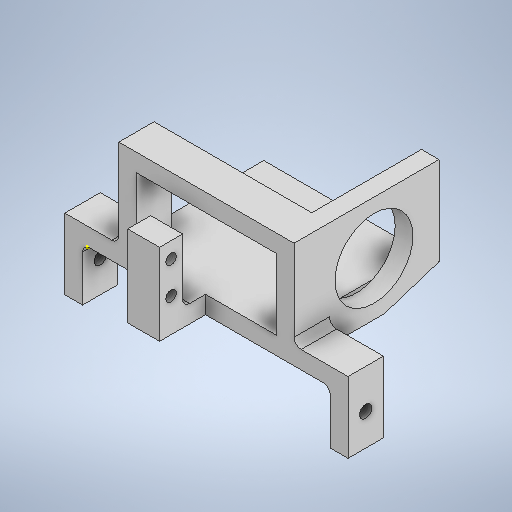
# Autodesk Inventor part: miau miau ggua gua loro loro
Saved by Autodesk Inventor 2025.2 (Build 292293000, 293)
## iProperties
Created: 2025-04-23
Part Number: miau miau ggua gua loro loro
Material: Generic
Document SubType Name: Modeling
Designer: maqmat
Density: 1 g/cm^3
Appearance: Default
Author: maqmat
Autodesk Inventor part; units mm, degrees
ref_plane "YZ Plane" through (0, 0, 0) normal (1, 0, 0) x (0, 1, 0)
ref_plane "XZ Plane" through (0, 0, 0) normal (0, 1, 0) x (-1, 0, 0)
ref_plane "XY Plane" through (0, 0, 0) normal (0, 0, 1) x (1, 0, 0)
sketch "Sketch1" plane through (0, 0, 0) normal (0, 1, 0) x (-1, 0, 0)
  line L0 (1.443, 4.6996) -> (-68.557, 4.6996)
  line L1 (-68.557, 4.6996) -> (-68.557, -5.3004)
  line L2 (-68.557, -5.3004) -> (1.443, -5.3004)
  line L3 (1.443, -5.3004) -> (1.443, 4.6996)
  line L4 (-68.557, 4.6996) -> (-73.557, 4.6996)
  line L5 (-73.557, 4.6996) -> (-73.557, -5.3004)
  line L6 (-73.557, -5.3004) -> (-68.557, -5.3004)
  line L7 (1.443, 4.6996) -> (6.443, 4.6996)
  line L8 (6.443, 4.6996) -> (6.443, -5.3004)
  line L9 (6.443, -5.3004) -> (1.443, -5.3004)
  point P0 (0, 0)
  dimension "d0" = 70
  dimension "d1" = 10
  dimension "d2" = 5
  dimension "d3" = 5
  constraints: 20 end point, 5 perpendicular, 3 horizontal, 2 parallel
  measures "d0" distance of L2.end L1.end
  measures "d1" distance of L1.end L0.end
  measures "d2" distance of L0.end L4.end
  measures "d3" distance of L0.start L7.end
extrude "Extrusion1" add sketch "Sketch1" against normal blind 15 contours L7 L8 L9 L3 | L1 L6 L5 L4
extrude "Extrusion2" add sketch "Sketch1" along normal blind 5
sketch "Sketch2" plane through (0, 5, 0) normal (0, 1, 0) x (1, 0, 0)
  line L0 (-6.443, 5.3004) -> (-6.443, -4.6996) projected
  line L1 (73.557, 5.3004) -> (-6.443, 5.3004) projected
  line L2 (-6.443, -4.6996) -> (-6.443, 5.3004)
  line L3 (33.557, 0.3004) -> (53.307, 0.3004)
  line L4 (33.557, 0.3004) -> (13.807, 0.3004)
  line L5 (73.557, 5.9707) -> (73.557, 3.1355)
  line L6 (73.557, 3.1355) -> (-6.443, 3.1355)
  line L7 (73.557, -4.6996) -> (73.557, -2.1996)
  line L8 (73.557, -2.1996) -> (-6.443, -2.1996)
  line L9 (53.307, 3.1355) -> (53.307, -2.1996)
  line L10 (13.807, 3.1355) -> (13.807, -2.1996)
  line L11 (13.807, 3.1355) -> (8.807, 3.1355)
  line L12 (8.807, 3.1355) -> (8.807, -2.1996)
  line L13 (53.307, 3.1355) -> (58.307, 3.1355)
  line L14 (58.307, 3.1355) -> (58.307, -2.1996)
  point P0 (0, 0)
  dimension "d8" = 19.75
  dimension "d9" = 19.75
  dimension "d10" = 5
  dimension "d11" = 5
  constraints: 26 end point, 11 point on line, 6 perpendicular, 1 vertical
  measures "d8" distance of L3.start L3.end
  measures "d9" distance of L3.start L4.end
  measures "d10" distance of L10.start L11.end
  measures "d11" distance of L9.start L13.end
extrude "Extrusion3" add sketch "Sketch2" along normal blind 25 contours L6 L10 L8 L12 | L6 L9 L3 L4 L10 | L14 L8 L9 L6 | L10 L4 L3 L9 L8
sketch "Sketch3" plane through (8.807, 5, 2.1996) normal (0, 0, 1) x (1, 0, 0)
  line L0 (0, 0) -> (0, 25) projected
  line L1 (0, 12.5) -> (5, 12.5)
  line L2 (49.5513, 12.5) -> (44.5513, 12.5)
  line L3 (49.5, 25) -> (0, 25) projected
  line L4 (5, 25) -> (5, -0.0015)
  line L5 (64.75, 0) -> (-15.25, 0) projected
  line L6 (44.5513, 0) -> (44.5513, 25)
  line L7 (5, -0.0015) -> (5, 19.9985)
  line L8 (5, 19.9985) -> (44.5513, 19.9985)
  point P0 (-8.807, -5)
  point P1 (5, 0)
  dimension "d14" = 5
  dimension "d15" = 5
  dimension "d16" = 20
  constraints: 12 end point, 7 point on line, 2 perpendicular, 1 horizontal, 1 midpoint, 1 vertical
  measures "d14" distance of L1.start L1.end
  measures "d15" distance of L2.start L2.end
  measures "d16" distance of L4.end L7.end
extrude "Extrusion4" cut sketch "Sketch3" against normal blind 25 contours L4 L8 L6 L5
sketch "Sketch4" plane through (-1.443, -15, 4.6996) normal (1, 0, 0) x (0, 0, -1)
  line L0 (10, 20) -> (0, 20) projected
  line L1 (5, 20) -> (5, 15)
  line L2 (5, 15) -> (10, 15)
  line L3 (10, 0) -> (10, 20) projected
  line L4 (0, 0) -> (0, 20) projected
  line L5 (0, 15) -> (10, 15)
  line L6 (5, 15) -> (5, 9)
  circle A0 centre (5, 9) radius 1.75
  point P0 (4.6996, 15)
  dimension "d20" = 6
  dimension "d21" = 3.5
  constraints: 8 end point, 3 perpendicular, 2 point on line, 1 centre point, 1 coincident, 1 midpoint, 1 vertical
  measures "d20" distance of L1.end L6.end
  measures "d21" diameter of A0
extrude "Extrusion5" add sketch "Sketch4" along normal blind 5.5 contours A0
mirror "Mirror1" about plane through (0, 0, 0) normal (1, 0, 0) of "Extrusion5"
pattern_linear "Rectangular Pattern1" count 2 spacing 64.5 along (1, 0, 0) of "Extrusion5"
sketch "Sketch5" plane through (68.557, -15, 4.6996) normal (0, 0, 1) x (1, 0, 0)
  point P0 (-68.557, 15)
sketch "Sketch6" plane through (68.557, -15, 4.6996) normal (0, 0, 1) x (1, 0, 0)
  line L0 (-54.75, 20) -> (-54.75, 39.9985) projected
  line L1 (-54.75, 21.2054) -> (-54.75, 18.7459)
  line L2 (-75, 20) -> (5, 20) projected
  line L3 (-54.75, 20) -> (-44.25, 20)
  line L4 (-44.25, 22.427) -> (-44.25, 20)
  line L5 (-58.8793, 22.427) -> (-58.8793, 20)
  line L6 (-54.75, 20) -> (-59.75, 20) projected
  line L7 (-58.8793, 22.427) -> (-44.25, 22.427)
  line L8 (-70, 15) -> (0, 15) projected
  line L9 (-44.25, 15) -> (-44.25, 20)
  line L10 (-44.25, 15) -> (-35.25, 15)
  line L11 (-35.25, 15) -> (-35.25, 20)
  line L12 (-35.25, 20) -> (-44.25, 20)
  line L13 (-44.25, 20) -> (-44.25, 15)
  line L14 (-15.1987, 22.427) -> (-15.1987, 20)
  line L15 (-10.25, 20) -> (-15.1987, 20) projected
  line L16 (-15.1987, 20) -> (-24.1987, 20)
  line L17 (-24.1987, 20) -> (-24.1987, 15)
  line L18 (-15.1987, 20) -> (-15.1987, 15)
  line L19 (-24.1987, 15) -> (-15.1987, 15)
  point P0 (-68.557, 15)
  dimension "d28" = 10.5
  dimension "d29" = 9
  dimension "d30" = 9
  constraints: 30 end point, 7 point on line, 4 vertical, 2 horizontal, 2 parallel, 2 perpendicular, 1 collinear, 4 other
  measures "d28" distance of L3.start L3.end
  measures "d29" distance of L12.end L11.end
  measures "d30" distance of L14.end L16.end
extrude "Extrusion6" add sketch "Sketch6" along normal blind 6 contours L2 L18 L8 L17
extrude "Extrusion7" add sketch "Sketch6" along normal blind 13 contours L2 L11 L8 L9
sketch "Sketch7" plane through (0, 5, 0) normal (0, 1, 0) x (1, 0, 0)
  line L0 (44.3582, -4.6996) -> (44.3582, -10.6996) projected
  line L1 (53.3582, -4.6996) -> (53.3582, -10.6996) projected
  line L2 (44.3582, -4.6996) -> (53.3582, -4.6996)
  line L3 (53.3582, -4.6996) -> (53.3582, -10.6996)
  line L4 (53.3582, -10.6996) -> (44.3582, -10.6996)
  line L5 (44.3582, -10.6996) -> (44.3582, -4.6996)
  point P0 (0, 0)
  constraints: 8 end point, 2 parallel, 1 horizontal, 1 perpendicular
extrude "Extrusion8" cut sketch "Sketch7" against normal blind 13
sketch "Sketch8" plane through (0, 5, 0) normal (0, 1, 0) x (1, 0, 0)
  line L0 (24.307, -4.6996) -> (24.307, -17.6996) projected
  line L1 (33.307, -4.6996) -> (33.307, -17.6996) projected
  line L2 (24.307, -4.6996) -> (33.307, -4.6996)
  line L3 (33.307, -4.6996) -> (33.307, -17.6996)
  line L4 (33.307, -17.6996) -> (24.307, -17.6996)
  line L5 (24.307, -17.6996) -> (24.307, -4.6996)
  line L6 (24.307, -11.1996) -> (33.307, -11.1996)
  point P0 (0, 0)
  constraints: 10 end point, 3 perpendicular, 2 midpoint, 1 collinear
extrude "Extrusion9" add sketch "Sketch8" along normal blind 18 contours L6 L1 L4 L0
sketch "Sketch9" plane through (24.307, 0, 4.6996) normal (-1, 0, 0) x (0, 0, 1)
  line L0 (0, 5) -> (6.5, 5) projected
  line L1 (6.5, 5) -> (13, 5)
  line L2 (13, 0) -> (13, 23) projected
  line L3 (9.75, 5) -> (9.75, 23)
  line L4 (6.5, 23) -> (13, 23) projected
  line L5 (9.75, 14) -> (6.5, 14)
  line L6 (6.5, 5) -> (6.5, 23) projected
  line L7 (9.75, 14) -> (13, 14)
  line L8 (9.75, 23) -> (9.75, 14)
  line L9 (9.75, 5) -> (9.75, 14)
  circle A0 centre (9.75, 9.5) radius 1.5
  circle A1 centre (9.75, 18.5) radius 1.5
  point P0 (-4.6996, 0)
  dimension "d39" = 3
  dimension "d40" = 3
  constraints: 12 end point, 6 midpoint, 2 centre point, 2 point on line, 1 collinear, 1 horizontal, 1 perpendicular
  measures "d39" diameter of A0
  measures "d40" diameter of A1
extrude "Extrusion10" cut sketch "Sketch9" against normal blind 10 contours A0 L3 | L3 A0 | A1 L3 | L3 A1
thread "Thread1" size "M3x0.5" class "6H" standard "ANSI Metric M Profile" full length
thread "Thread2" size "M3x0.5" class "6H" standard "ANSI Metric M Profile" full length
sketch "Sketch11" plane through (-6.443, -15, -5.3004) normal (-1, 0, 0) x (0, 0, 1)
  circle A0 centre (5, 9) radius 1.75 projected
  circle A1 centre (5, 9) radius 1.75
  point P0 (5.3004, 15)
  constraints: 1 centre point, 1 coincident
extrude "Extrusion12" cut sketch "Sketch11" against normal blind 20
sketch "Sketch12" plane through (73.557, -15, 4.6996) normal (1, 0, 0) x (0, 0, -1)
  circle A0 centre (5, 9) radius 1.75 projected
  circle A1 centre (5, 9) radius 1.75
  point P0 (4.6996, 15)
  constraints: 1 centre point, 1 coincident
extrude "Extrusion13" cut sketch "Sketch12" against normal blind 20
sketch "Sketch13" plane through (8.807, 30, 2.1996) normal (0, 0, 1) x (1, 0, 0)
  line L0 (64.75, -25) -> (-15.25, -25) projected
  line L1 (49.5, 0) -> (0, 0) projected
  line L2 (44.4862, -25) -> (49.5, -25)
  line L3 (49.5, -25) -> (49.5, 0)
  line L4 (49.5, 0) -> (44.4862, 0)
  line L5 (44.4862, 0) -> (44.4862, -25)
  line L6 (0, -25) -> (0, 0) projected
  line L7 (5, -5.0015) -> (44.5513, -5.0015) projected
  line L8 (0, -25) -> (5, -25)
  line L9 (5, -25) -> (5, -5.0015)
  line L10 (5, -5.0015) -> (0, -5.0015)
  line L11 (0, -5.0015) -> (0, -25)
  line L12 (0, 0) -> (49.5, 0)
  line L13 (49.5, 0) -> (49.5, -5.0015)
  line L14 (49.5, -5.0015) -> (0, -5.0015)
  line L15 (0, -5.0015) -> (0, 0)
  point P0 (-8.807, -30)
  point P1 (44.4862, -5.0015)
  constraints: 24 end point, 6 parallel, 3 horizontal, 3 perpendicular, 2 point on line
extrude "Extrusion14" add sketch "Sketch13" along normal blind 2.5 contours L0 L5 L7 L14 L3 | L14 L7 L5 L1 L3 | L0 L6 L10 L9 | L7 L10 L6 L1 L5
sketch "Sketch14" plane through (58.307, 30, -3.1355) normal (0, 0, -1) x (-1, 0, 0)
  line L0 (49.5, -25) -> (49.5, 0) projected
  line L1 (0, 0) -> (49.5, 0) projected
  line L2 (49.5, -25) -> (44.5333, -25)
  line L3 (44.5333, -25) -> (44.5333, 0)
  line L4 (44.5333, 0) -> (49.5, 0)
  line L5 (49.5, 0) -> (49.5, -25)
  line L6 (4.9487, -25) -> (4.9487, -5.0015) projected
  line L7 (0, -25) -> (0, 0) projected
  line L8 (4.9487, -25) -> (0, -25)
  line L9 (0, -25) -> (0, 0)
  line L10 (0, 0) -> (4.9487, 0)
  line L11 (4.9487, 0) -> (4.9487, -25)
  line L12 (44.5, -5.0015) -> (5.0138, -5.0015) projected
  line L13 (0, 0) -> (44.5, 0)
  line L14 (44.5, 0) -> (44.5, -5.0015)
  line L15 (44.5, -5.0015) -> (0, -5.0015)
  line L16 (0, -5.0015) -> (0, 0)
  point P0 (58.307, -30)
  constraints: 24 end point, 6 parallel, 3 horizontal, 3 perpendicular, 1 point on line
extrude "Extrusion15" add sketch "Sketch14" along normal blind 2.12
sketch "Sketch15" plane through (58.307, 30, -5.2555) normal (0, 0, -1) x (-1, 0, 0)
  line L0 (0, -25) -> (0, 0) projected
  line L1 (5.0138, -5.0015) -> (5.0138, -25) projected
  line L2 (0, -25) -> (5.0138, -25)
  line L3 (5.0138, -25) -> (5.0138, -5.0015)
  line L4 (5.0138, -5.0015) -> (0, -5.0015)
  line L5 (0, -5.0015) -> (0, -25)
  point P0 (58.307, -30)
  constraints: 8 end point, 2 parallel, 1 horizontal, 1 perpendicular
extrude "Extrusion16" add sketch "Sketch15" along normal blind 31
sketch "Sketch16" plane through (58.307, 5, 4.6996) normal (1, 0, 0) x (0, 0, -1)
  line L0 (9.9551, 0) -> (9.9551, 19.9985) projected
  line L1 (9.9551, 9.9993) -> (22.5751, 9.9993)
  circle A0 centre (22.5751, 9.9993) radius 11
  point P0 (4.6996, -5)
  dimension "d59" = 12.62
  dimension "d60" = 22
  constraints: 2 end point, 1 centre point, 1 coincident, 1 horizontal, 1 midpoint
  measures "d59" distance of L1.start L1.end
  measures "d60" diameter of A0
sketch "Sketch17" plane through (58.307, 30, -5.2555) normal (0, 0, -1) x (-1, 0, 0)
  line L0 (4.9487, -5.0015) -> (4.9487, -25) projected
  line L1 (0, -25) -> (0, 0) projected
  line L2 (4.9487, -5.0015) -> (0, -5.0015)
  line L3 (0, -5.0015) -> (0, 0)
  line L4 (0, 0) -> (4.9487, 0)
  line L5 (4.9487, 0) -> (4.9487, -5.0015)
  point P0 (58.307, -30)
  constraints: 8 end point, 2 parallel, 1 horizontal, 1 perpendicular
extrude "Extrusion17" add sketch "Sketch17" along normal blind 31
sketch "Sketch18" plane through (73.557, -15, -5.3004) normal (0, 0, -1) x (-1, 0, 0)
  line L0 (15.25, 20) -> (15.25, 45) projected
  line L1 (5, 15) -> (75, 15) projected
  line L2 (15.25, 20) -> (20.263, 20)
  line L3 (20.263, 20) -> (20.263, 15)
  line L4 (20.263, 15) -> (15.25, 15)
  line L5 (15.25, 15) -> (15.25, 20)
  point P0 (73.557, 15)
  constraints: 8 end point, 2 parallel, 1 horizontal, 1 perpendicular, 1 point on line
extrude "Extrusion18" add sketch "Sketch18" along normal blind 31
sketch "Sketch19" plane through (58.307, 5, 4.6996) normal (1, 0, 0) x (0, 0, -1)
  line L0 (10, -5) -> (41, -5) projected
  line L1 (40.9551, 25) -> (40.9551, 0) projected
  line L2 (25.5, -5) -> (40.9551, 0)
  line L3 (25.5, -5) -> (41, -5)
  line L4 (41, -5) -> (41, 0) projected
  line L5 (41, 0) -> (41, -5)
  line L6 (41, -5) -> (25.5, -5)
  line L7 (41, 0) -> (25.5, -5)
  line L8 (41, -5) -> (41, 0)
  point P0 (4.6996, -5)
  constraints: 12 end point, 3 collinear, 1 midpoint, 1 perpendicular
extrude "Extrusion19" cut sketch "Sketch19" against normal blind 11
extrude "Extrusion20" cut sketch "Sketch16" against normal blind 11
sketch "Sketch20" plane through (53.2939, 0, -5.3004) normal (-1, 0, 0) x (0, 0, 1)
  line L0 (-30.9551, 5) -> (-17.1593, 5) projected
  line L1 (-30.9551, 5) -> (-15.5, 0)
  line L2 (-31, 5) -> (-15.5, 0) projected
  line L3 (0, 0) -> (-15.5, 0) projected
  line L4 (0, 5) -> (0, 0) projected
  line L5 (0, 0) -> (0, 5)
  line L6 (0, 5) -> (-30.9551, 5)
  point P0 (5.3004, 0)
  constraints: 7 end point, 1 collinear, 1 perpendicular
extrude "Extrusion21" add sketch "Sketch20" along normal blind 44.5
sketch "Sketch21" plane through (8.807, 5, 4.6996) normal (-1, 0, 0) x (0, 0, 1)
  line L0 (0, 0) -> (0, 19.9985) projected
  line L1 (-9.9551, 25) -> (-9.9551, 19.9985) projected
  line L2 (0, 0) -> (-9.9551, 0)
  line L3 (-9.9551, 0) -> (-9.9551, 25)
  line L4 (-9.9551, 25) -> (0, 25)
  line L5 (0, 25) -> (0, 0)
  point P0 (-4.6996, -5)
  constraints: 8 end point, 2 parallel, 1 horizontal, 1 perpendicular
extrude "Extrusion22" add sketch "Sketch21" against normal blind 5
fillet "Fillet4" radius 2 5 edges at (28.807, 5, 11.1996) (-1.443, 0, -0.3004) (68.557, 0, -0.3004) (58.307, 5, -0.3004) (8.807, 5, -0.278)
thread "Thread3" size "M3.5x0.6" class "6H" standard "ANSI Metric M Profile" full length
thread "Thread4" size "M3.5x0.6" class "6H" standard "ANSI Metric M Profile" full length
body "Solid1"
